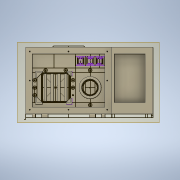
# Autodesk Inventor part: authentication panel v1.1
Saved by Autodesk Inventor 2022 (Build 260153000, 153)
## iProperties
Created: 2022-05-25
Part Number: authentication panel v1.1
Material: Generic
Document SubType Name: Modeling
Designer: alecw
Density: 1 g/cm^3
Appearance: Default
Author: alecw
Autodesk Inventor part; units mm, degrees
ref_plane "YZ Plane" through (0, 0, 0) normal (1, 0, 0) x (0, 1, 0)
ref_plane "XZ Plane" through (0, 0, 0) normal (0, 1, 0) x (-1, 0, 0)
ref_plane "Backplate Depth" through (0, 0, -3.2) normal (0, 0, 1) x (1, 0, 0)
sketch "Sketch2" plane through (0, 0, 0) normal (0, 0, 1) x (1, 0, 0)
  line L0 (0, 0) -> (45, 0)
  line L1 (45, 0) -> (45, 65)
  line L2 (45, 65) -> (0, 65)
  line L3 (0, 65) -> (0, 0)
  line L4 (0, 0) -> (-8.8, 0)
  line L5 (-8.8, 0) -> (-12, 0)
  line L6 (-12, 0) -> (-42, 0)
  line L7 (-42, 0) -> (-54.8, 0)
  line L8 (-54.8, 0) -> (-99.5, 0)
  line L9 (-99.5, 0) -> (-105.9, 0)
  line L10 (-105.9, 0) -> (-114.7, 0)
  line L11 (-114.7, 0) -> (-114.7, 40.1)
  line L12 (-114.7, 40.1) -> (0, 40.1)
  line L13 (-114.7, 0) -> (0, 0)
  line L14 (-105.9, 0) -> (-105.9, 40.1)
  line L15 (-8.8, 40.1) -> (-8.8, 0)
  line L16 (-48.4, 0) -> (-8.8, 0)
  line L17 (0, 65) -> (-114.7, 65)
  line L18 (-114.7, 65) -> (-114.7, 40.1)
  line L19 (45, 0) -> (48.2, 0)
  line L20 (0, 65) -> (0, 68.2)
  line L21 (0, 68.2) -> (48.2, 68.2)
  line L22 (48.2, 68.2) -> (48.2, 0)
  line L23 (-54.8, 0) -> (-48.4, 0)
  line L24 (-42, 0) -> (-48.4, 0)
  line L25 (-48.4, 0) -> (-48.4, 40.1)
  line L26 (-105.9, 40.1) -> (-105.9, 33.7)
  line L27 (-105.9, 40.1) -> (-93.1, 40.1)
  line L28 (-105.9, 0) -> (-48.4, 0)
  line L29 (-99.5, 0) -> (-88.19, 0)
  line L30 (-88.19, 0) -> (-79.22, 0)
  line L31 (-54.8, 0) -> (-54.8, 40.1)
  line L32 (-99.5, 0) -> (-99.5, 40.1)
  line L33 (-54.8, 40.1) -> (-56.9213, 37.9787)
  line L34 (-54.8, 40.1) -> (-51.8, 40.1) construction
  line L35 (-56.9213, 37.9787) -> (-54.8, 35.8574)
  line L36 (-56.9213, 37.9787) -> (-59.0426, 40.1)
  line L37 (-54.8, 0) -> (-57.6284, 2.8284)
  line L38 (-54.8, 0) -> (-50.8, 0) construction
  line L39 (-99.5, 40.1) -> (-95.9645, 36.5645)
  line L40 (-99.5, 40.1) -> (-94.5, 40.1) construction
  line L41 (-95.9645, 36.5645) -> (-92.4289, 40.1)
  line L42 (-95.9645, 36.5645) -> (-99.5, 33.0289)
  line L43 (-99.5, 0) -> (-95.9645, 3.5355)
  line L44 (-99.5, 0) -> (-94.5, 0) construction
  line L45 (-95.9645, 3.5355) -> (-92.4289, 0)
  line L46 (-95.9645, 3.5355) -> (-99.5, 7.0711)
  line L47 (-48.4, 0) -> (-48.4, -6.4)
  line L48 (-48.4, -6.4) -> (-105.9, -6.4)
  line L49 (-105.9, -6.4) -> (-105.9, 0)
  line L50 (-105.9, 40.1) -> (-105.9, 46.5)
  line L51 (-48.4, 40.1) -> (-48.4, 46.5)
  line L52 (-48.4, 46.5) -> (-105.9, 46.5)
  line L53 (-88.19, 0) -> (-86.59, 0)
  line L54 (-88.19, 0) -> (-89.79, 0)
  line L55 (-89.79, 0) -> (-86.59, 0)
  line L56 (-86.59, 0) -> (-86.59, 40.1)
  line L57 (-86.59, 40.1) -> (-89.79, 40.1)
  line L58 (-89.79, 40.1) -> (-89.79, 0)
  line L59 (-80.82, 40.1) -> (-80.82, 0)
  line L60 (-77.62, 0) -> (-77.62, 40.1)
  line L61 (-71.85, 40.1) -> (-71.85, 0)
  line L62 (-68.65, 0) -> (-68.65, 40.1)
  line L63 (-62.88, 40.1) -> (-62.88, 0)
  line L64 (-59.68, 0) -> (-59.68, 40.1)
  line L65 (0, 0) -> (0, -6.4)
  line L66 (0, -6.4) -> (0, -15.2)
  line L67 (-114.7, 0) -> (-114.7, -6.4)
  line L68 (-114.7, -6.4) -> (-114.7, -15.2)
  line L69 (-114.7, -15.2) -> (0, -15.2)
  line L70 (0, -15.2) -> (48.2, -15.2)
  line L71 (48.2, -15.2) -> (48.2, 0)
  line L72 (-28.6, 40.1) -> (-28.6, 0)
  circle A0 centre (-28.6, 20.05) radius 9.5
  circle A1 centre (-28.6, 20.05) radius 10.5
  line L73 (-28.6, 29.55) -> (-27.303, 29.4611)
  line L74 (-27.303, 29.4611) -> (-27.2345, 30.4608)
  line L75 (-28.6, 29.55) -> (-29.897, 29.4611)
  line L76 (-29.897, 29.4611) -> (-29.9655, 30.4608)
  line L77 (-105.9, 46.5) -> (-114.7, 46.5)
  line L78 (-105.9, -6.4) -> (-114.7, -6.4)
  line L79 (-48.4, -6.4) -> (0, -6.4)
  line L80 (-28.6, 20.05) -> (-35, 20.05)
  line L81 (-28.6, 20.05) -> (-22.2, 20.05)
  circle A2 centre (-28.6, 20.05) radius 14.7
  line L82 (-77.62, 40.1) -> (-71.85, 40.1)
  line L83 (-88.19, 40.1) -> (-92.19, 40.1)
  line L84 (-92.19, 40.1) -> (-93.79, 40.1)
  line L85 (-74.735, 0) -> (-74.735, 40.1)
  line L86 (-92.135, 38.25) -> (-57.335, 38.25)
  line L87 (-57.335, 38.25) -> (-57.335, 1.85)
  line L88 (-57.335, 1.85) -> (-92.135, 1.85)
  line L89 (-92.135, 1.85) -> (-92.135, 38.25)
  line L90 (-92.135, 38.25) -> (-57.335, 1.85) construction
  line L91 (-57.335, 38.25) -> (-92.135, 1.85) construction
  line L92 (-74.735, 38.25) -> (-74.735, 40.1)
  line L93 (-18.1, 20.05) -> (-17.1, 20.05)
  circle A3 centre (-28.6, 20.05) radius 11.5
  line L94 (-17.1, 20.05) -> (-13.9, 20.05)
  line L95 (-54.8, 40.1) -> (-48.4, 40.1)
  line L96 (-89.79, 38.25) -> (-86.59, 38.25)
  line L97 (-59.68, 38.25) -> (-62.88, 38.25)
  line L98 (-92.135, 20.05) -> (-57.335, 20.05)
  line L99 (-57.6284, 2.8284) -> (-54.8, 5.6569)
  line L100 (-57.6284, 2.8284) -> (-60.4569, 0)
  line L101 (-99.5, 20.05) -> (-105.9, 20.05)
  circle A4 centre (-102.7, 20.05) radius 0.9
  line L102 (-54.8, 20.05) -> (-48.4, 20.05)
  circle A5 centre (-51.6, 20.05) radius 0.9
  line L103 (0, -15.2) -> (0, -20)
  line L104 (0, -20) -> (-114.7, -20)
  line L105 (-114.7, -20) -> (-114.7, -15.2)
  line L106 (-88.19, 40.1) -> (-88.19, 43.3)
  circle A6 centre (-88.19, 43.3) radius 0.9
  circle A7 centre (-61.28, 43.3) radius 0.9
  line L107 (-102.7, 20.05) -> (-102.7, 0)
  circle A8 centre (-102.7, 10.025) radius 0.9
  circle A9 centre (-102.7, 30.075) radius 0.9
  circle A10 centre (-51.6, 30.075) radius 0.9
  circle A11 centre (-51.6, 10.025) radius 0.9
  line L108 (0, -20) -> (48.2, -20)
  line L109 (48.2, -20) -> (48.2, -15.2)
  line L110 (0, 65) -> (0, 73.8)
  line L111 (0, 73.8) -> (-114.7, 73.8)
  line L112 (-114.7, 73.8) -> (-114.7, 65)
  line L113 (-105.9, -20) -> (-105.9, 73.8)
  line L114 (-8.8, -20) -> (-8.8, 73.8)
  line L115 (-28.6, 40.1) -> (-48.4, 40.1)
  line L116 (-28.6, 40.1) -> (-8.8, 40.1)
  line L117 (-48.4, 46.5) -> (-28.6, 46.5)
  line L118 (-28.6, 46.5) -> (-8.8, 46.5)
  line L119 (-28.6, 46.5) -> (-28.6, 65)
  line L120 (-25.4, 52.55) -> (-31.8, 52.55)
  line L121 (-31.8, 52.55) -> (-31.8, 58.95)
  line L122 (-31.8, 58.95) -> (-25.4, 58.95)
  line L123 (-25.4, 58.95) -> (-25.4, 52.55)
  line L124 (-25.4, 52.55) -> (-31.8, 58.95) construction
  line L125 (-31.8, 52.55) -> (-25.4, 58.95) construction
  line L126 (-24.1, 51.25) -> (-33.1, 51.25)
  line L127 (-33.1, 51.25) -> (-33.1, 60.25)
  line L128 (-33.1, 60.25) -> (-24.1, 60.25)
  line L129 (-24.1, 60.25) -> (-24.1, 51.25)
  line L130 (-24.1, 51.25) -> (-33.1, 60.25) construction
  line L131 (-33.1, 51.25) -> (-24.1, 60.25) construction
  line L132 (-25.4, 52.55) -> (-25.4, 51.25)
  line L133 (-31.8, 52.55) -> (-31.8, 51.25)
  circle A12 centre (-88.19, 43.3) radius 2.4
  circle A13 centre (-61.28, 43.3) radius 2.4
  circle A14 centre (-51.6, 30.075) radius 2.4
  circle A15 centre (-51.6, 20.05) radius 2.4
  circle A16 centre (-102.7, 10.025) radius 2.4
  circle A17 centre (-102.7, 20.05) radius 2.4
  circle A18 centre (-102.7, 30.075) radius 2.4
  line L134 (-114.7, -20) -> (-114.7, -22.4)
  line L135 (-114.7, -22.4) -> (-117.1, -22.4)
  line L136 (-114.7, -15.2) -> (-114.7, -12.8)
  line L137 (-114.7, -12.8) -> (-112.3, -12.8)
  line L138 (0, 73.8) -> (-2.4, 73.8)
  line L139 (-2.4, 73.8) -> (-2.4, 71.4)
  line L140 (-112.3, -12.8) -> (-112.3, 71.4)
  line L141 (-112.3, 71.4) -> (-2.4, 71.4)
  line L142 (-2.4, 71.4) -> (-2.4, -12.8)
  line L143 (-2.4, -12.8) -> (-112.3, -12.8)
  line L144 (-2.4, -15.2) -> (-2.4, -12.8)
  line L145 (-28.6, -6.4) -> (-28.6, 0)
  circle A19 centre (-28.6, -3.2) radius 2.4
  circle A20 centre (-28.6, -3.2) radius 0.9
  line L146 (-28.6, 40.1) -> (-28.6, 46.5)
  circle A21 centre (-28.6, 43.3) radius 0.9
  circle A22 centre (-28.6, 43.3) radius 2.4
  line L147 (-105.9, 65) -> (-105.9, 71.4)
  circle A23 centre (-109.1, 68.2) radius 0.9
  circle A24 centre (-109.1, 68.2) radius 2
  line L148 (-8.8, 65) -> (-2.4, 65)
  line L149 (-8.8, -6.4) -> (-8.8, -12.8)
  line L150 (-105.9, 65) -> (-112.3, 65)
  line L151 (-105.9, 65) -> (-105.9, 71.4)
  line L152 (-105.9, 68.2) -> (-109.1, 68.2)
  line L153 (-109.1, 65) -> (-109.1, 68.2)
  line L154 (-105.9, -6.4) -> (-105.9, -12.8)
  circle A25 centre (-57.35, 68.2) radius 2
  circle A26 centre (-57.35, 68.2) radius 0.9
  circle A27 centre (-5.6, 68.2) radius 2
  circle A28 centre (-5.6, 68.2) radius 0.9
  circle A29 centre (-109.1, -9.6) radius 2
  circle A30 centre (-109.1, -9.6) radius 0.9
  circle A31 centre (-57.35, -9.6) radius 2
  circle A32 centre (-57.35, -9.6) radius 0.9
  circle A33 centre (-5.6, -9.6) radius 2
  circle A34 centre (-5.6, -9.6) radius 0.9
  line L155 (-105.9, -6.4) -> (-105.9, 65)
  line L156 (-105.9, 29.3) -> (-112.3, 29.3)
  circle A35 centre (-109.1, 29.3) radius 2
  circle A36 centre (-109.1, 29.3) radius 0.9
  circle A37 centre (-5.6, 29.3) radius 0.9
  circle A38 centre (-5.6, 29.3) radius 2
  line L157 (-105.9, 29.3) -> (-105.9, 65)
  line L158 (-8.8, 65) -> (-105.9, 65)
  line L159 (-57.35, 65) -> (-109.1, 65)
  circle A39 centre (-109.1, 68.2) radius 1.6
  circle A40 centre (-97.6, 68.2) radius 1.6
  circle A41 centre (-86.1, 68.2) radius 1.6
  circle A42 centre (-74.6, 68.2) radius 1.6
  circle A43 centre (-63.1, 68.2) radius 1.6
  circle A44 centre (-51.6, 68.2) radius 1.6
  circle A45 centre (-40.1, 68.2) radius 1.6
  circle A46 centre (-28.6, 68.2) radius 1.6
  circle A47 centre (-17.1, 68.2) radius 1.6
  circle A48 centre (-109.1, 57.0857) radius 1.6
  circle A49 centre (-109.1, 45.9714) radius 1.6
  circle A50 centre (-109.1, 34.8571) radius 1.6
  circle A51 centre (-109.1, 23.7429) radius 1.6
  circle A52 centre (-109.1, 12.6286) radius 1.6
  circle A53 centre (-109.1, 1.5143) radius 1.6
  line L160 (-57.35, 65) -> (-57.35, 71.4)
  circle A54 centre (-97.6, -9.6) radius 1.6
  circle A55 centre (-86.1, -9.6) radius 1.6
  circle A56 centre (-74.6, -9.6) radius 1.6
  circle A57 centre (-63.1, -9.6) radius 1.6
  circle A58 centre (-51.6, -9.6) radius 1.6
  circle A59 centre (-40.1, -9.6) radius 1.6
  circle A60 centre (-28.6, -9.6) radius 1.6
  circle A61 centre (-17.1, -9.6) radius 1.6
  circle A62 centre (-5.6, 57.0857) radius 1.6
  circle A63 centre (-5.6, 45.9714) radius 1.6
  circle A64 centre (-5.6, 34.8571) radius 1.6
  circle A65 centre (-5.6, 23.7429) radius 1.6
  circle A66 centre (-5.6, 12.6286) radius 1.6
  circle A67 centre (-5.6, 1.5143) radius 1.6
  line L161 (-48.4, 46.5) -> (-48.4, 65)
  line L162 (-92.135, 38.25) -> (-92.985, 38.25)
  line L163 (-92.985, 38.25) -> (-92.985, 39.1)
  line L164 (-56.485, 1) -> (-92.985, 1)
  line L165 (-92.985, 1) -> (-92.985, 39.1)
  line L166 (-92.985, 39.1) -> (-56.485, 39.1)
  line L167 (-56.485, 39.1) -> (-56.485, 1)
  line L168 (-56.485, 1) -> (-92.985, 39.1) construction
  line L169 (-92.985, 1) -> (-56.485, 39.1) construction
  line L170 (-92.985, 39.1) -> (-92.985, 40.1)
  line L171 (-92.985, 40.1) -> (-93.985, 40.1)
  line L172 (-55.485, 0) -> (-93.985, 0)
  line L173 (-93.985, 0) -> (-93.985, 40.1)
  line L174 (-93.985, 40.1) -> (-55.485, 40.1)
  line L175 (-55.485, 40.1) -> (-55.485, 0)
  line L176 (-55.485, 0) -> (-93.985, 40.1) construction
  line L177 (-93.985, 0) -> (-55.485, 40.1) construction
  line L178 (48.2, -20) -> (53.2, -20)
  line L179 (53.2, -20) -> (53.2, 68.2)
  line L180 (53.2, 68.2) -> (48.2, 68.2)
  line L181 (53.2, -20) -> (55.2, -20)
  line L182 (55.2, -20) -> (55.2, 68.2)
  line L183 (55.2, 68.2) -> (53.2, 68.2)
  line L184 (53.2, 65) -> (55.2, 65)
  line L185 (53.2, -20) -> (53.2, -16.8)
  line L186 (53.2, -16.8) -> (55.2, -16.8)
  line L187 (-8.8, -20) -> (-105.9, -20)
  line L188 (-105.9, -20) -> (-101.9, -20)
  line L189 (-57.35, -20) -> (-57.35, -15.2)
  line L190 (-101.9, -20) -> (-101.4, -20)
  line L191 (-101.4, -20) -> (-93.4, -20)
  line L192 (-93.4, -20) -> (-93.4, -15.2)
  line L193 (-101.9, -20) -> (-101.9, -15.2)
  line L194 (-101.4, -20) -> (-101.4, -15.2)
  line L195 (-93.4, -20) -> (-92.9, -20)
  line L196 (-92.9, -20) -> (-84.9, -20)
  line L197 (-84.9, -20) -> (-84.9, -15.2)
  line L198 (-8.8, -20) -> (-12.8, -20)
  line L199 (-12.8, -20) -> (-13.3, -20)
  line L200 (-13.3, -20) -> (-21.3, -20)
  line L201 (-21.3, -20) -> (-21.3, -15.2)
  line L202 (-12.8, -20) -> (-12.8, -15.2)
  line L203 (-13.3, -20) -> (-13.3, -15.2)
  line L204 (-21.3, -20) -> (-21.8, -20)
  line L205 (-21.8, -20) -> (-29.8, -20)
  line L206 (-29.8, -20) -> (-29.8, -15.2)
  line L207 (-57.35, 73.8) -> (-57.35, 75.8)
  line L208 (-57.35, 75.8) -> (-77.35, 75.8)
  line L209 (-77.35, 75.8) -> (-79.35, 73.8)
  line L210 (-77.35, 75.8) -> (-74.5216, 75.8) construction
  line L211 (-57.35, 75.8) -> (-37.35, 75.8)
  line L212 (-37.35, 75.8) -> (-35.35, 73.8)
  line L213 (0, 73.8) -> (55.2, 73.8)
  line L214 (55.2, 73.8) -> (55.2, 68.2)
  line L215 (0, 73.8) -> (0.5, 73.8)
  line L216 (0.5, 73.8) -> (0.5, -20)
  line L217 (53.2, 68.2) -> (53.2, 73.8)
  line L218 (48.2, -15.2) -> (55.2, -15.2)
  line L219 (-92.9, -20) -> (-92.9, -15.2)
  line L220 (-21.8, -20) -> (-21.8, -15.2)
  line L221 (0.5, -15.2) -> (0.5, -12)
  line L222 (0.5, -12) -> (48.2, -12)
  line L223 (0.5, -15.2) -> (0.5, -12)
  line L224 (0.5, -12) -> (48.2, -12)
  line L225 (45, 0) -> (45, -15.2)
  line L226 (45, 68.2) -> (45, 65)
  line L227 (48.2, 65) -> (45, 65)
  line L228 (0.5, -15.2) -> (3.7, -15.2)
  line L229 (3.7, -15.2) -> (3.7, 65)
  line L230 (48.2, 68.2) -> (48.2, 73.8)
  line L231 (45, 68.2) -> (45, 73.8)
  line L232 (45, -15.2) -> (45, -20)
  line L233 (3.7, -15.2) -> (3.7, -20)
  line L234 (3.7, 65) -> (3.7, 73.8)
  line L235 (48.2, -12) -> (55.2, -12)
  line L236 (55.2, 65) -> (48.2, 65)
  line L237 (-35, 20.05) -> (-35, 13.0293)
  line L238 (-35, 20.05) -> (-35, 27.0707)
  line L239 (-22.2, 20.05) -> (-22.2, 27.0707)
  line L240 (-22.2, 20.05) -> (-22.2, 13.0293)
  line L241 (0, -6.4) -> (55.2, -6.4)
  line L242 (0, 0) -> (55.2, 0)
  line L243 (-35, 27.0707) -> (-35, 33.2837)
  line L244 (-22.2, 27.0707) -> (-22.2, 33.2837)
  line L245 (-27.303, 10.6389) -> (-27.2345, 9.6392)
  line L246 (-29.897, 10.6389) -> (-29.9655, 9.6392)
  line L247 (-35, 20.05) -> (-35, 6.8163)
  line L248 (-22.2, 20.05) -> (-22.2, 6.8163)
  line L249 (-99.5, 33.0289) -> (-101.5, 33.0289)
  line L250 (-92.4289, 40.1) -> (-92.4289, 42.1)
  line L251 (-92.4289, 42.1) -> (-101.5, 42.1)
  line L252 (-101.5, 42.1) -> (-101.5, 33.0289)
  line L253 (-99.5, 7.0711) -> (-101.5, 7.0711)
  line L254 (-92.4289, 0) -> (-92.4289, -2)
  line L255 (-92.4289, -2) -> (-101.5, -2)
  line L256 (-101.5, -2) -> (-101.5, 7.0711)
  line L257 (-54.8, 5.6569) -> (-52.8, 5.6569)
  line L258 (-60.4569, 0) -> (-60.4569, -2)
  line L259 (-60.4569, -2) -> (-52.8, -2)
  line L260 (-52.8, -2) -> (-52.8, 5.6569)
  line L261 (-59.0426, 40.1) -> (-59.0426, 42.1)
  line L262 (-54.8, 35.8574) -> (-52.8, 35.8574)
  line L263 (-52.8, 35.8574) -> (-52.8, 42.1)
  line L264 (-52.8, 42.1) -> (-59.0426, 42.1)
  line L265 (-28.6, 52.55) -> (-30.1, 52.55)
  line L266 (-30.1, 52.55) -> (-30.1, 51.25)
  line L267 (-28.6, 52.55) -> (-27.1, 52.55)
  line L268 (-27.1, 52.55) -> (-27.1, 51.25)
  line L269 (-2.4, 29.3) -> (-2.4, 32.5)
  line L270 (-2.4, 32.5) -> (-8.8, 32.5)
  line L271 (-2.4, 29.3) -> (-2.4, 26.1)
  line L272 (-2.4, 26.1) -> (-8.8, 26.1)
  line L273 (-27.1, 58.95) -> (-27.1, 60.25)
  line L274 (-30.1, 58.95) -> (-30.1, 60.25)
  line L275 (-31.8, 58.95) -> (-31.8, 62.15)
  line L276 (-31.8, 62.15) -> (-35, 62.15)
  line L277 (-22.2, 49.35) -> (-35, 49.35)
  line L278 (-35, 49.35) -> (-35, 62.15)
  line L279 (-35, 62.15) -> (-22.2, 62.15)
  line L280 (-22.2, 62.15) -> (-22.2, 49.35)
  line L281 (-22.2, 49.35) -> (-35, 62.15) construction
  line L282 (-35, 49.35) -> (-22.2, 62.15) construction
  line L283 (-31.8, 58.95) -> (-32.1, 58.95)
  line L284 (-32.1, 58.95) -> (-32.1, 59.25)
  line L285 (-25.1, 52.25) -> (-32.1, 52.25)
  line L286 (-32.1, 52.25) -> (-32.1, 59.25)
  line L287 (-32.1, 59.25) -> (-25.1, 59.25)
  line L288 (-25.1, 59.25) -> (-25.1, 52.25)
  line L289 (-25.1, 52.25) -> (-32.1, 59.25) construction
  line L290 (-32.1, 52.25) -> (-25.1, 59.25) construction
  line L291 (-28.6, 55.75) -> (-28.6, 52.55)
  line L292 (-44.6, 52.55) -> (-38.2, 52.55)
  line L293 (-38.2, 52.55) -> (-38.2, 58.95)
  line L294 (-38.2, 58.95) -> (-44.6, 58.95)
  line L295 (-44.6, 58.95) -> (-44.6, 52.55)
  line L296 (-44.6, 52.55) -> (-38.2, 58.95) construction
  line L297 (-38.2, 52.55) -> (-44.6, 58.95) construction
  line L298 (-45.9, 51.25) -> (-36.9, 51.25)
  line L299 (-36.9, 51.25) -> (-36.9, 60.25)
  line L300 (-36.9, 60.25) -> (-45.9, 60.25)
  line L301 (-45.9, 60.25) -> (-45.9, 51.25)
  line L302 (-45.9, 51.25) -> (-36.9, 60.25) construction
  line L303 (-36.9, 51.25) -> (-45.9, 60.25) construction
  line L304 (-44.6, 52.55) -> (-44.6, 51.25)
  line L305 (-38.2, 52.55) -> (-38.2, 51.25)
  line L306 (-41.4, 52.55) -> (-39.9, 52.55)
  line L307 (-39.9, 52.55) -> (-39.9, 51.25)
  line L308 (-41.4, 52.55) -> (-42.9, 52.55)
  line L309 (-42.9, 52.55) -> (-42.9, 51.25)
  line L310 (-42.9, 58.95) -> (-42.9, 60.25)
  line L311 (-39.9, 58.95) -> (-39.9, 60.25)
  line L312 (-38.2, 58.95) -> (-38.2, 62.15)
  line L313 (-38.2, 62.15) -> (-35, 62.15)
  line L314 (-47.8, 49.35) -> (-35, 49.35)
  line L315 (-35, 62.15) -> (-47.8, 62.15)
  line L316 (-47.8, 62.15) -> (-47.8, 49.35)
  line L317 (-47.8, 49.35) -> (-35, 62.15) construction
  line L318 (-35, 49.35) -> (-47.8, 62.15) construction
  line L319 (-38.2, 58.95) -> (-37.9, 58.95)
  line L320 (-37.9, 58.95) -> (-37.9, 59.25)
  line L321 (-44.9, 52.25) -> (-37.9, 52.25)
  line L322 (-37.9, 52.25) -> (-37.9, 59.25)
  line L323 (-37.9, 59.25) -> (-44.9, 59.25)
  line L324 (-44.9, 59.25) -> (-44.9, 52.25)
  line L325 (-44.9, 52.25) -> (-37.9, 59.25) construction
  line L326 (-37.9, 52.25) -> (-44.9, 59.25) construction
  line L327 (-41.4, 55.75) -> (-41.4, 52.55)
  line L328 (-15.8, 46.5) -> (-15.8, 65)
  line L329 (-19, 52.55) -> (-12.6, 52.55)
  line L330 (-12.6, 52.55) -> (-12.6, 58.95)
  line L331 (-12.6, 58.95) -> (-19, 58.95)
  line L332 (-19, 58.95) -> (-19, 52.55)
  line L333 (-19, 52.55) -> (-12.6, 58.95) construction
  line L334 (-12.6, 52.55) -> (-19, 58.95) construction
  line L335 (-20.3, 51.25) -> (-11.3, 51.25)
  line L336 (-11.3, 51.25) -> (-11.3, 60.25)
  line L337 (-11.3, 60.25) -> (-20.3, 60.25)
  line L338 (-20.3, 60.25) -> (-20.3, 51.25)
  line L339 (-20.3, 51.25) -> (-11.3, 60.25) construction
  line L340 (-11.3, 51.25) -> (-20.3, 60.25) construction
  line L341 (-19, 52.55) -> (-19, 51.25)
  line L342 (-12.6, 52.55) -> (-12.6, 51.25)
  line L343 (-15.8, 52.55) -> (-14.3, 52.55)
  line L344 (-14.3, 52.55) -> (-14.3, 51.25)
  line L345 (-15.8, 52.55) -> (-17.3, 52.55)
  line L346 (-17.3, 52.55) -> (-17.3, 51.25)
  line L347 (-17.3, 58.95) -> (-17.3, 60.25)
  line L348 (-14.3, 58.95) -> (-14.3, 60.25)
  line L349 (-12.6, 58.95) -> (-12.6, 62.15)
  line L350 (-12.6, 62.15) -> (-9.4, 62.15)
  line L351 (-22.2, 49.35) -> (-9.4, 49.35)
  line L352 (-9.4, 49.35) -> (-9.4, 62.15)
  line L353 (-9.4, 62.15) -> (-22.2, 62.15)
  line L354 (-22.2, 49.35) -> (-9.4, 62.15) construction
  line L355 (-9.4, 49.35) -> (-22.2, 62.15) construction
  line L356 (-12.6, 58.95) -> (-12.3, 58.95)
  line L357 (-12.3, 58.95) -> (-12.3, 59.25)
  line L358 (-19.3, 52.25) -> (-12.3, 52.25)
  line L359 (-12.3, 52.25) -> (-12.3, 59.25)
  line L360 (-12.3, 59.25) -> (-19.3, 59.25)
  line L361 (-19.3, 59.25) -> (-19.3, 52.25)
  line L362 (-19.3, 52.25) -> (-12.3, 59.25) construction
  line L363 (-12.3, 52.25) -> (-19.3, 59.25) construction
  line L364 (-15.8, 55.75) -> (-15.8, 52.55)
  line L365 (-77.15, 46.5) -> (-77.15, 65)
  point P0 (-74.735, 20.05)
  point P1 (-74.735, 20.05)
  point P2 (-112.3, 0)
  point P3 (-8.8, 71.4)
  point P4 (0.5, 0)
  point P5 (53.2, -15.2)
  point P6 (-8.8, -15.2)
  point P7 (-105.9, -15.2)
  point P8 (3.7, 0)
  point P9 (53.2, 0)
  point P10 (-60.4569, 0)
  point P11 (-60.4569, 0)
  point P12 (-92.4289, 0)
  point P13 (-68.65, 38.25)
  point P14 (-71.85, 38.25)
  point P15 (-71.85, 1.85)
  point P16 (-68.65, 1.85)
  point P17 (-62.88, 1.85)
  point P18 (-59.68, 1.85)
  point P19 (-80.82, 1.85)
  point P20 (-77.62, 1.85)
  point P21 (-77.62, 38.25)
  point P22 (-80.82, 38.25)
  point P23 (-86.59, 38.25)
  point P24 (-89.79, 1.85)
  point P25 (-86.59, 1.85)
  point P26 (-92.4289, 0)
  point P27 (-60.4569, 0)
  dimension "d1" = 45
  dimension "d2" = 65
  dimension "d3" = 8.8
  dimension "d4" = 3.2
  dimension "d5" = 30
  dimension "d6" = 12.8
  dimension "d7" = 44.7
  dimension "d11" = 40.1
  dimension "d15" = 3.2
  dimension "d16" = 3.2
  dimension "d21" = 11.31
  dimension "d22" = 8.97
  dimension "d23" = 3
  dimension "d24" = 135
  dimension "d25" = 4
  dimension "d26" = 135
  dimension "d27" = 5
  dimension "d28" = 45
  dimension "d29" = 5
  dimension "d30" = 45
  dimension "d33" = 6.4
  dimension "d34" = 1.6
  dimension "d35" = 1.6
  dimension "d38" = 8.97
  dimension "d43" = 3.2
  dimension "d45" = 19
  dimension "d46" = 21
  dimension "d47" = 1.3
  dimension "d48" = 6.4
  dimension "d49" = 6.4
  dimension "d53" = 4
  dimension "d54" = 1.6
  dimension "d55" = 34.8
  dimension "d56" = 36.4
  dimension "d59" = 1
  dimension "d61" = 3.2
  dimension "d70" = 1.8
  dimension "d71" = 1.8
  dimension "d72" = 4.8
  dimension "d74" = 3.2
  dimension "d75" = 1.8
  dimension "d76" = 1.8
  dimension "d79" = 51.1
  dimension "d86" = 6.4
  dimension "d88" = 9
  dimension "d89" = 4.8
  dimension "d98" = 2.4
  dimension "d99" = 2.4
  dimension "d100" = 2.4
  dimension "d101" = 2.4
  dimension "d102" = 2.4
  dimension "d103" = 2.4
  dimension "d104" = 2.4
  dimension "d105" = 1.8
  dimension "d106" = 4
  dimension "d109" = 51.75
  dimension "d116" = 77.8
  dimension "d123" = 38.9
  dimension "d128" = 3.2
  dimension "d131" = 11.5
  dimension "d138" = 11.1143
  dimension "d143" = 0.85
  dimension "d144" = 0.85
  dimension "d145" = 1
  constraints: 728 end point, 139 point on line, 94 symmetric about line, 68 centre point, 66 perpendicular, 61 midpoint, 55 horizontal, 45 vertical, 37 parallel, 23 coincident, 19 collinear, 15 point on circle, 14 horizontal alignment, 12 equal radius, 5 equal length, 96 other
  measures "d1" distance of L2.end L1.end
  measures "d2" distance of L1.end L0.end
  measures "d3" distance of L0.start L4.end
  measures "d4" distance of L4.end L5.end
  measures "d5" distance of L5.end L6.end
  measures "d6" distance of L6.end L7.end
  measures "d7" distance of L7.end L8.end
  measures "d11" distance of L10.end L11.end
  measures "d15" distance of L0.end L19.end
  measures "d16" distance of L2.end L20.end
  measures "d21" distance of L8.end L29.end
  measures "d22" distance of L29.end L30.end
  measures "d23" distance of L31.end L33.end
  measures "d24" angle of L33 L34
  measures "d25" distance of L7.end L37.end
  measures "d26" angle of L38 L37
  measures "d27" distance of L32.end L39.end
  measures "d28" angle of L39 L40
  measures "d29" distance of L8.end L43.end
  measures "d30" angle of L44 L43
  measures "d33" distance of L25.end L51.end
  measures "d34" distance of L29.end L53.end
  measures "d35" distance of L29.end L54.end
  measures "d38" distance of L57.end L59.start
  measures "d43" distance between parallel lines of L56 L58
  measures "d45" diameter of A0
  measures "d46" diameter of A1
  measures "d47" distance of L73.start L73.end
  measures "d48" distance of L80.start L80.end
  measures "d49" distance of L80.start L81.end
  measures "d53" distance of L83.start L83.end
  measures "d54" distance of L83.end L84.end
  measures "d55" distance of L87.end L88.end
  measures "d56" distance of L86.end L87.end
  measures "d59" distance of L93.start L93.end
  measures "d61" distance of L94.start L94.end
  measures "d70" diameter of A4
  measures "d71" diameter of A5
  measures "d72" distance of L66.end L103.end
  measures "d74" distance of L83.start L106.end
  measures "d75" diameter of A6
  measures "d76" diameter of A8
  measures "d79" distance of A9.centre A10.centre
  measures "d86" distance of L121.end L122.end
  measures "d88" distance of L126.end L127.end
  measures "d89" diameter of A12
  measures "d98" distance of L104.end L134.end
  measures "d99" distance of L134.end L135.end
  measures "d100" distance of L68.end L136.end
  measures "d101" distance of L136.end L137.end
  measures "d102" distance of L110.end L138.end
  measures "d103" distance of L138.end L139.end
  measures "d104" distance of L144.start L142.end
  measures "d105" diameter of A23
  measures "d106" diameter of A24
  measures "d109" distance of L152.end A25.centre
  measures "d116" distance of L152.end A29.centre
  measures "d123" distance of L152.end A35.centre
  measures "d128" diameter of A39
  measures "d131" distance of A39.centre A40.centre
  measures "d138" distance of A39.centre A48.centre
  measures "d143" distance of L86.start L162.end
  measures "d144" distance of L162.end L163.end
  measures "d145" distance of L163.end L170.end
ref_plane "Face Plate Start" through (0, 0, 5) normal (0, 0, 1) x (1, 0, 0)
ref_plane "TPU Seal Start" through (0, 0, 4) normal (0, 0, 1) x (1, 0, 0)
ref_plane "Face Plate End" through (0, 0, 8.2) normal (0, 0, 1) x (1, 0, 0)
ref_plane "Cover Clearance" through (0, 0, 11.2) normal (0, 0, 1) x (1, 0, 0)
ref_plane "Cover End" through (0, 0, 13.6) normal (0, 0, 1) x (1, 0, 0)
extrude "backplate" add sketch "Sketch2" against normal up to surface (3.2 mm away) contours L3 L2 L216 L0 | L4 L142 L12 L3 | L65 L79 L142 L4 | L0 L216 L241 L65 | L216 L2 L229 L0 | L0 L229 L241 L216 | L12 L142 L17 L3 | L142 L79 L114 L4 A67 | L4 A67 L15 L272 L142 | L241 L216 L70 L66 | L66 L69 L144 L142 L79 | L229 L2 L1 L0 | L0 L225 L241 L229 | L216 L21 L234 L2 | L2 L20 L21 L216 | L241 L229 L222 L216 | L17 L142 L139 L111 L110 L20 | L142 L270 L15 L12 | L12 L114 L17 L142 | A67 L4 | L4 A67 | L272 L15 L270 L142 | L142 L143 L114 L79 | L1 L227 L22 L19 | L19 L71 L241 L225 | L241 L225 L222 L229 | L234 L21 L226 L2 | L216 L213 L234 L21 | L21 L110 L213 L216 | L222 L229 L70 L216 | L17 L114 L141 L142 | L15 L5 L6 L72 A2 L12 | L12 L146 A22 L118 L114 | L114 L143 L113 L48 L79 | L79 L145 A19 L6 L5 L114 | L144 L69 L114 L143 | L226 L21 L22 L227 | L242 L179 L241 L71 | L22 L236 L179 L242 | L241 L71 L222 L225 | L222 L225 L70 L229 | L234 L213 L231 L21 | L114 L118 L328 L351 L352 L350 L353 L17 | L17 L160 A25 L141 L114 | L141 L114 L111 L139 | L72 A2 L6 L7 L25 L12 | L12 L51 L117 L146 A22 | L79 L47 L7 L6 L145 A19 | L114 L69 L113 L143 | L231 L213 L230 L21 | L22 L180 L179 L236 | L241 L179 L235 L71 | L222 L71 L70 L225 | L328 L353 L279 L119 L17 | L141 L113 L111 L114 | L25 L102 A15 L31 L262 L263 L12 | L12 L263 L264 L261 L250 L251 L252 L50 L52 L51 | A2 L244 A3 L72 | L72 A3 L243 A2 | A22 L146 A21 | L146 A21 A22 | L118 L119 L277 L351 L328 | L48 L49 L9 L256 L255 L254 L8 L258 L259 L260 L7 L47 | A19 L145 A20 | L145 A20 A19 | L143 L140 L78 L113 | L113 L69 L68 L137 L143 | L230 L213 L217 L180 | L235 L179 L218 L71 | L119 L279 L276 L313 L315 L316 L314 L277 L117 L161 L17 | L353 L349 L337 L328 | L328 L337 L338 L335 L351 L280 L353 | L160 A25 L17 L113 L141 | L263 L262 L31 L12 | L12 L261 L264 L263 | L25 L7 L260 L257 L31 L102 A15 | L52 L365 L17 L161 | A3 L244 A1 L72 | L72 A1 L243 A3 | A2 L94 A3 L244 | L243 A3 L247 A2 | A21 L146 | L146 A21 | L328 L335 L336 L337 L349 L350 L352 L351 | L78 L140 L10 A53 L49 | A20 L145 | L145 A20 | L137 L68 L78 L140 | L279 L280 L277 L119 L126 L129 L128 | L119 L128 L275 L279 | L337 L348 L360 L328 | L328 L360 L347 L337 | L141 L140 L17 L112 L111 L113 | L113 L152 A24 L153 L17 L140 L141 | L160 A26 A25 | A25 L160 A26 | L33 L175 L12 | L31 L35 L175 L33 | A15 L102 A5 | L102 A5 A15 | L52 L113 L17 L365 | A1 L74 A0 L72 | L72 A0 L76 A1 | A3 L93 A1 L244 | L243 A1 L247 A3 | A2 L248 A3 L94 | L247 A3 L72 A2 | L277 L278 L276 L275 L128 L127 L126 L119 | L335 L346 L358 L328 | L328 L358 L344 L335 | L72 A3 L248 A2 | L260 L259 L258 L8 L7 | L7 L31 L257 L260 | L14 L101 A17 L107 A16 L9 | L10 A53 L140 L156 A35 L14 | L78 L67 L10 L140 | L128 L273 L287 L119 | L119 L287 L274 L128 | L360 L348 L331 L328 | L328 L331 L347 L360 | L337 L349 L360 L348 | L347 L360 L361 L358 L341 L335 L338 L337 | L337 L336 L335 L342 L358 L359 L357 L360 L349 | L113 L17 L153 A24 L152 | L160 A26 | A26 L160 | L175 L33 L167 L166 L36 L12 | L31 L99 L175 L35 | L175 L35 L167 L33 | A5 L102 | L102 A5 | L50 L12 L140 L77 A49 | L77 A49 L140 L17 L113 | L73 A0 L239 L81 L72 | L75 A0 | A0 L73 | L72 L80 L238 A0 L75 | A1 L244 A0 L74 | L76 A0 L243 A1 | A3 L248 A1 L93 | A1 L248 A0 L244 | L247 A1 L72 A3 | L243 A0 L247 A1 | L126 L266 L285 L119 | L119 L285 L268 L126 | L314 L316 L315 L313 L278 | L358 L346 L329 L328 | L328 L329 L344 L358 | L335 L341 L358 L346 | L344 L358 L342 L335 | L72 A1 L248 A3 | L37 L175 L99 L31 | L8 L175 L37 | L107 A16 A17 L101 L32 L253 L256 L9 | A53 L10 | L10 A53 | L14 L12 L252 L249 L32 L101 A17 | L10 L11 L12 L140 | L287 L273 L122 L119 | L119 L122 L274 L287 | L274 L287 L275 L128 | L128 L129 L126 L132 L285 L288 L287 L273 | L275 L287 L284 L286 L285 L133 L126 L127 L128 | L331 L330 L329 L328 | L328 L329 L332 L331 | L360 L349 L331 L348 | L347 L331 L332 L341 L358 L361 L360 | L360 L357 L356 L349 | L152 A39 L153 A24 | A24 L153 A39 L152 | L140 L77 L18 L17 | L36 L166 L64 L12 | L175 L99 L167 L35 | L167 L35 L33 | L33 L36 L166 L167 | L14 L156 A35 L140 L12 | A49 L77 | L77 A49 | L81 L240 A0 L72 | L72 A0 L237 L80 | A0 L240 L239 | L247 A0 L246 A1 | L238 L237 A0 | L285 L266 L120 L119 | L119 L120 L268 L285 | L268 L285 L132 L126 | L126 L133 L285 L266 | L358 L341 L329 L346 | L344 L329 L342 L358 | A1 L246 A0 L72 | L72 A0 L245 A1 | L8 L64 L100 L164 L167 L37 L175 | L37 L167 L99 L175 | L256 L253 L32 L9 | L9 L8 L254 L255 L256 | A16 L107 A8 | L107 A8 A16 | A17 L101 A4 | L101 A4 L107 A17 | L122 L123 L120 L119 | L119 L120 L121 L122 | L274 L122 L275 L287 | L287 L288 L285 L132 L123 L122 L273 | L275 L283 L284 L287 | L356 L359 L358 L342 L330 | A39 L153 A23 L152 | L152 A23 L153 A39 | L140 L12 L18 L77 | L64 L166 L63 L12 | L36 L35 L167 L99 L87 L86 L64 L166 | L252 L251 L250 L12 | L12 L32 L249 L252 | A1 L245 A0 L248 | L268 L120 L132 L285 | L285 L133 L120 L266 | L8 L100 L64 | L167 L164 L100 L88 L87 L37 | L37 L87 L99 L167 | L8 L63 L164 L64 L100 | L43 L45 L173 L8 | L32 L46 L43 | A8 L107 | L107 A8 | A35 L156 A36 | L156 A36 A35 | A4 L101 | L101 L107 A4 | A17 L107 A4 L101 | L121 L133 L285 L286 L283 | L152 L153 A23 | A23 L153 L152 | L63 L166 L62 L12 | L64 L86 L63 L166 | L39 L42 L32 | L12 L173 L41 L39 | L64 L164 L100 | L87 L88 L100 L37 | L37 L99 L87 | L8 L62 L164 L63 | L173 L45 L8 | L32 L42 L41 L173 L45 L46 | A36 L156 | L156 A36 | L101 A4 L107 | L62 L166 L61 L12 | L63 L86 L62 L166 | L86 L87 L98 L64 | L64 L98 L63 L86 | L99 L100 L88 L64 L98 L87 | L12 L170 L41 L173 | L164 L63 L88 L64 | L64 L88 L100 L164 | L8 L61 L164 L62 | L164 L62 L88 L63 | L45 L173 L41 L170 L163 L165 L164 L58 L8 | L61 L166 L85 L12 | L62 L86 L61 L166 | L63 L98 L62 L86 | L64 L88 L63 L98 | L41 L170 L12 | L12 L58 L166 L170 L41 | L8 L85 L164 L61 | L164 L61 L88 L62 | L88 L62 L98 L63 | L58 L164 L56 L8 | L85 L166 L60 L12 | L61 L86 L85 L166 | L62 L98 L61 L86 | L8 L60 L164 L85 | L164 L85 L88 L61 | L88 L61 L98 L62 | L164 L165 L162 L89 L88 L58 | L58 L88 L56 L164 | L60 L166 L59 L12 | L85 L86 L60 L166 | L61 L98 L85 L86 | L166 L58 L86 L162 L163 | L12 L56 L166 L58 | L8 L59 L164 L60 | L164 L60 L88 L85 | L88 L85 L98 L61 | L56 L164 L59 L8 | L88 L89 L98 L58 | L58 L98 L56 L88 | L56 L88 L59 L164 | L59 L166 L56 L12 | L60 L86 L59 L166 | L85 L98 L60 L86 | L166 L56 L86 L58 | L164 L59 L88 L60 | L88 L60 L98 L85 | L98 L89 L86 L58 | L58 L86 L56 L98 | L56 L98 L59 L88 | L59 L86 L56 L166 | L60 L98 L59 L86 | L88 L59 L98 L60 | L56 L86 L59 L98 | A6 | A7 | A9 | A10 | A11 | A12 | A13 | A14 | A18 | A27 | A28 | A29 | A30 | A31 | A32 | A33 | A34 | A37 | A38 | A40 | A41 | A42 | A43 | A44 | A45 | A46 | A47 | A48 | A50 | A51 | A52 | A54 | A55 | A56 | A57 | A58 | A59 | A60 | A61 | A62 | A63 | A64 | A65 | A66 | L295 L294 L293 L292 | L304 L321 L324 L323 L310 L294 L295 | L292 L309 L321 L304 | L292 L307 L321 L309 | L321 L309 L298 L304 | L304 L298 L301 L300 L310 L323 L324 L321 | L321 L307 L298 L309 | L310 L323 L311 L294 | L292 L305 L321 L307 | L321 L305 L298 L307 | L311 L323 L312 L294 | L310 L300 L311 L323 | L293 L319 L322 L321 L305 | L321 L322 L320 L323 L312 L300 L299 L298 L305 | L312 L323 L320 L319 | L311 L300 L312 L323
extrude "enclosure walls" add sketch "Sketch2" along normal up to surface (5 mm away) contours L3 L2 L216 L0 | L4 L142 L12 L3 | L65 L79 L142 L4 | L0 L216 L241 L65 | L216 L2 L229 L0 | L0 L229 L241 L216 | L12 L142 L17 L3 | L142 L79 L114 L4 A67 | L4 A67 L15 L272 L142 | L241 L216 L70 L66 | L66 L69 L144 L142 L79 | L0 L225 L241 L229 | L216 L21 L234 L2 | L2 L20 L21 L216 | L241 L229 L222 L216 | L17 L142 L139 L111 L110 L20 | L142 L270 L15 L12 | L12 L114 L17 L142 | A67 L4 | L4 A67 | L272 L15 L270 L142 | L142 L143 L114 L79 | L1 L227 L22 L19 | L19 L71 L241 L225 | L241 L225 L222 L229 | L234 L21 L226 L2 | L216 L213 L234 L21 | L21 L110 L213 L216 | L222 L229 L70 L216 | L17 L114 L141 L142 | L114 L143 L113 L48 L79 | L144 L69 L114 L143 | L226 L21 L22 L227 | L242 L179 L241 L71 | L22 L236 L179 L242 | L241 L71 L222 L225 | L222 L225 L70 L229 | L234 L213 L231 L21 | L17 L160 A25 L141 L114 | L141 L114 L111 L139 | L114 L69 L113 L143 | L231 L213 L230 L21 | L22 L180 L179 L236 | L241 L179 L235 L71 | L242 L182 L241 L179 | L179 L184 L182 L242 | L222 L71 L70 L225 | L141 L113 L111 L114 | L143 L140 L78 L113 | L113 L69 L68 L137 L143 | L230 L213 L217 L180 | L179 L183 L182 L184 | L235 L179 L218 L71 | L241 L182 L235 L179 | L160 A25 L17 L113 L141 | L78 L140 L10 A53 L49 | L137 L68 L78 L140 | L217 L213 L214 L183 | L235 L182 L218 L179 | L141 L140 L17 L112 L111 L113 | L113 L152 A24 L153 L17 L140 L141 | L160 A26 A25 | A25 L160 A26 | L10 A53 L140 L156 A35 L14 | L78 L67 L10 L140 | L113 L17 L153 A24 L152 | L160 A26 | A26 L160 | L50 L12 L140 L77 A49 | L77 A49 L140 L17 L113 | A53 L10 | L10 A53 | L10 L11 L12 L140 | L152 A39 L153 A24 | A24 L153 A39 L152 | L140 L77 L18 L17 | L14 L156 A35 L140 L12 | A49 L77 | L77 A49 | A39 L153 A23 L152 | L152 A23 L153 A39 | L140 L12 L18 L77 | A35 L156 A36 | L156 A36 A35 | L152 L153 A23 | A23 L153 L152 | A36 L156 | L156 A36 | A27 | A28 | A29 | A30 | A31 | A32 | A33 | A34 | A37 | A38 | A40 | A41 | A42 | A43 | A44 | A45 | A46 | A47 | A48 | A50 | A51 | A52 | A54 | A55 | A56 | A57 | A58 | A59 | A60 | A61 | A62 | A63 | A64 | A65 | A66
extrude "enclosure hinges" add sketch "Sketch2" against normal blind 4.8 from surface at 8.2 contours L114 L104 L202 L69 | L69 L193 L104 L113 | L220 L104 L206 L69 | L69 L197 L104 L219
extrude "fingerprint seal support" add sketch "Sketch2" along normal up to surface (4 mm away) contours A2 L244 A3 L72 | L72 A3 L243 A2 | A2 L94 A3 L244 | L243 A3 L247 A2 | A2 L248 A3 L94 | L247 A3 L72 A2 | L72 A3 L248 A2
extrude "wire pass through" cut sketch "Sketch2" along normal blind 2 contours L3 L2 L216 L0 | L4 L142 L12 L3 | L216 L2 L229 L0 | L12 L142 L17 L3 | L4 A67 L15 L272 L142 | L142 L270 L15 L12 | L12 L114 L17 L142 | L4 A67 | L272 L15 L270 L142 | L1 L227 L22 L19 | L22 L236 L179 L242 | L179 L184 L182 L242 | A2 L244 A3 L72 | L72 A3 L243 A2 | A3 L244 A1 L72 | L72 A1 L243 A3 | A1 L74 A0 L72 | L72 A0 L76 A1 | A1 L244 A0 L74 | L76 A0 L243 A1 | A37 | A38 | A62 | A63 | A64 | A65 | A66 picked at (-5.8995, 1.9409)
chamfer "Chamfer1" distance 2 angle 45 2 edges at (55.2, -7.6, 0) (55.2, 69.4, 0)
extrude "face plate screw holes" cut sketch "Sketch2" against normal up to surface (5 mm away) from surface at 5 contours L160 A26 | A26 L160 | L152 L153 A23 | A23 L153 L152 | A36 L156 | L156 A36 | A28 | A30 | A32 | A34 | A37
extrude "keypad holders" add sketch "Sketch2" along normal up to surface (5 mm away) contours L263 L262 L31 L12 | L12 L261 L264 L263 | L33 L175 L12 | L31 L35 L175 L33 | L260 L259 L258 L8 L7 | L7 L31 L257 L260 | L175 L33 L167 L166 L36 L12 | L175 L35 L167 L33 | L37 L175 L99 L31 | L8 L175 L37 | L167 L35 L33 | L33 L36 L166 L167 | L8 L64 L100 L164 L167 L37 L175 | L37 L167 L99 L175 | L256 L253 L32 L9 | L9 L8 L254 L255 L256 | L252 L251 L250 L12 | L12 L32 L249 L252 | L8 L100 L64 | L167 L164 L100 L88 L87 L37 | L37 L87 L99 L167 | L43 L45 L173 L8 | L32 L46 L43 | L39 L42 L32 | L12 L173 L41 L39 | L87 L88 L100 L37 | L37 L99 L87 | L173 L45 L8 | L64 L98 L63 L86 | L12 L170 L41 L173 | L64 L88 L63 L98 | L41 L170 L12 | L62 L98 L61 L86 | L88 L61 L98 L62 | L58 L98 L56 L88 | L58 L86 L56 L98 | L60 L98 L59 L86 | L88 L59 L98 L60
extrude "keypad holder clearance from face plate" cut sketch "Sketch2" against normal blind 0.5 from surface at 5 contours L263 L262 L31 L12 | L12 L261 L264 L263 | L260 L259 L258 L8 L7 | L7 L31 L257 L260 | L256 L253 L32 L9 | L9 L8 L254 L255 L256 | L252 L251 L250 L12 | L12 L32 L249 L252
extrude "Extrusion9" cut sketch "Sketch2" against normal blind 2.6 from surface at 5 contours L33 L175 L12 | L31 L35 L175 L33 | L175 L33 L167 L166 L36 L12 | L175 L35 L167 L33 | L37 L175 L99 L31 | L8 L175 L37 | L167 L35 L33 | L33 L36 L166 L167 | L8 L64 L100 L164 L167 L37 L175 | L37 L167 L99 L175 | L8 L100 L64 | L167 L164 L100 L88 L87 L37 | L37 L87 L99 L167 | L43 L45 L173 L8 | L32 L46 L43 | L39 L42 L32 | L12 L173 L41 L39 | L87 L88 L100 L37 | L37 L99 L87 | L173 L45 L8 | L64 L98 L63 L86 | L12 L170 L41 L173 | L64 L88 L63 L98 | L41 L170 L12 | L62 L98 L61 L86 | L88 L61 L98 L62 | L58 L98 L56 L88 | L58 L86 L56 L98 | L60 L98 L59 L86 | L88 L59 L98 L60
ref_plane "RFID Cover Start" through (0, 0, 12) normal (0, 0, 1) x (1, 0, 0)
extrude "Extrusion10" add sketch "Sketch2" along normal up to surface (7 mm away) from surface at 5 contours L216 L2 L229 L0 | L0 L229 L241 L216 | L0 L225 L241 L229 | L216 L21 L234 L2 | L241 L229 L222 L216 | L1 L227 L22 L19 | L19 L71 L241 L225 | L241 L225 L222 L229 | L234 L21 L226 L2 | L216 L213 L234 L21 | L222 L229 L70 L216 | L226 L21 L22 L227 | L242 L179 L241 L71 | L22 L236 L179 L242 | L241 L71 L222 L225 | L222 L225 L70 L229 | L234 L213 L231 L21 | L231 L213 L230 L21 | L22 L180 L179 L236 | L241 L179 L235 L71 | L242 L182 L241 L179 | L179 L184 L182 L242 | L222 L71 L70 L225 | L230 L213 L217 L180 | L179 L183 L182 L184 | L235 L179 L218 L71 | L241 L182 L235 L179 | L217 L213 L214 L183 | L235 L182 L218 L179
body "Solid1"
